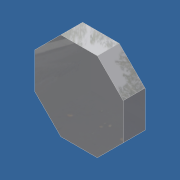
# Autodesk Inventor part: Oktagon
Saved by Autodesk Inventor 2018.2 (Build 222227000, 227)
## iProperties
Created: 2018-10-01
Part Number: Oktagon
Material: Kst - PVC (rigid/white)
Document SubType Name: Modeling
Designer: N.Grubert
Density: 1.38 g/cm^3
Appearance: Glatt - weiß
Author: N.Grubert
Fläche: 0 cm²
Gewicht: 0 g
Material: geeigneten Werkstoff auswählen !
Dateiname: P:\INVENTOR\Inventor 2018\Templates\ILT\Norm.ipt
Bez_eng: bolt
Bez_french: boulon
Autodesk Inventor part; units mm, degrees
ref_plane "YZ Plane" through (0, 0, 0) normal (1, 0, 0) x (0, 1, 0)
ref_plane "XZ Plane" through (0, 0, 0) normal (0, 1, 0) x (-1, 0, 0)
ref_plane "XY Plane" through (0, 0, 0) normal (0, 0, 1) x (1, 0, 0)
sketch "Skizze4" plane through (0, 0, 0) normal (0, 1, 0) x (-1, 0, 0)
  line L0 (77.8517, 0) -> (-77.8517, 0) construction
  line L1 (0, -77.8517) -> (0, 77.8517) construction
  line L2 (27, 37.5) -> (-27, 37.5) construction
  line L3 (-27, 37.5) -> (-27, -37.5) construction
  line L4 (-27, -37.5) -> (27, -37.5) construction
  line L5 (27, -37.5) -> (27, 37.5) construction
  line L6 (55.6084, -23.0337) -> (23.0337, -55.6084)
  line L7 (23.0337, -55.6084) -> (-23.0337, -55.6084)
  line L8 (-23.0337, -55.6084) -> (-55.6084, -23.0337)
  line L9 (-55.6084, -23.0337) -> (-55.6084, 23.0337)
  line L10 (-55.6084, 23.0337) -> (-23.0337, 55.6084)
  line L11 (-23.0337, 55.6084) -> (23.0337, 55.6084)
  line L12 (23.0337, 55.6084) -> (55.6084, 23.0337)
  line L13 (55.6084, 23.0337) -> (55.6084, -23.0337)
  line L14 (53.1084, -21.9982) -> (21.9982, -53.1084)
  line L15 (21.9982, -53.1084) -> (-21.9982, -53.1084)
  line L16 (-21.9982, -53.1084) -> (-53.1084, -21.9982)
  line L17 (-53.1084, -21.9982) -> (-53.1084, 21.9982)
  line L18 (-53.1084, 21.9982) -> (-21.9982, 53.1084)
  line L19 (-21.9982, 53.1084) -> (21.9982, 53.1084)
  line L20 (21.9982, 53.1084) -> (53.1084, 21.9982)
  line L21 (53.1084, 21.9982) -> (53.1084, -21.9982)
  point P0 (0, 0)
  point P1 (0, 0)
  dimension "d4" = 75
  dimension "d5" = 54
  dimension "d6" = 10
  dimension "d7" = 2.5
  constraints: 40 end point, 2 parallel, 1 coincident, 1 horizontal, 1 perpendicular, 27 other
  measures "d4" distance between parallel lines of L4 L2
  measures "d5" distance between parallel lines of L3 L5
  measures "d6" distance from line of L6 L4.end
  measures "d7" distance between parallel lines of L13 L21
extrude "Extrusion2" add sketch "Skizze4" along normal blind 25
sketch "Skizze5" plane through (0, 0, 0) normal (0, -1, 0) x (1, 0, 0)
  line L0 (21.9982, -53.1084) -> (-21.9982, -53.1084) projected
  line L1 (-21.9982, -53.1084) -> (-53.1084, -21.9982) projected
  line L2 (-53.1084, -21.9982) -> (-53.1084, 21.9982) projected
  line L3 (-53.1084, 21.9982) -> (-21.9982, 53.1084) projected
  line L4 (-21.9982, 53.1084) -> (21.9982, 53.1084) projected
  line L5 (21.9982, 53.1084) -> (53.1084, 21.9982) projected
  line L6 (53.1084, 21.9982) -> (53.1084, -21.9982) projected
  line L7 (53.1084, -21.9982) -> (21.9982, -53.1084) projected
  line L8 (-55.6084, -23.0337) -> (-23.0337, -55.6084) projected
  line L9 (-23.0337, -55.6084) -> (23.0337, -55.6084) projected
  line L10 (23.0337, -55.6084) -> (55.6084, -23.0337) projected
  line L11 (55.6084, -23.0337) -> (55.6084, 23.0337) projected
  line L12 (55.6084, 23.0337) -> (23.0337, 55.6084) projected
  line L13 (23.0337, 55.6084) -> (-23.0337, 55.6084) projected
  line L14 (-23.0337, 55.6084) -> (-55.6084, 23.0337) projected
  line L15 (-55.6084, 23.0337) -> (-55.6084, -23.0337) projected
  point P0 (0, 0)
extrude "Extrusion3" add sketch "Skizze5" along normal blind 2.5 contours L0 L1 L2 L3 L4 L5 L6 L7 | L15 L14 L13 L12 L11 L10 L9 L8
